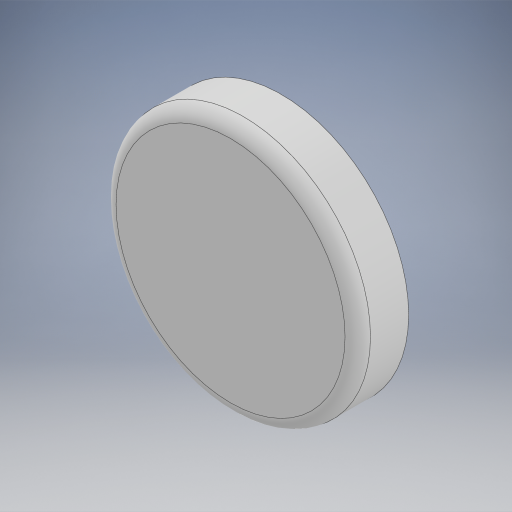
# Autodesk Inventor part: Brikker
Saved by Autodesk Inventor 2024 (Build 280153000, 153)
## iProperties
Created: 2024-03-15
Part Number: Brikker
Material: Generic
Document SubType Name: Modeling
Designer: fluen
Density: 1 g/cm^3
Appearance: Default
Author: fluen
## iProperties of the stored document Brikker_3DPrint.ipt
Created: 2024-04-12
Part Number: Brikker_3DPrint
Material: Generic
Document SubType Name: Modeling
Designer: Faber
Density: 1 g/cm^3
Appearance: Default
Author: Faber
Autodesk Inventor part; units mm, degrees
ref_plane "YZ Plane" through (0, 0, 0) normal (1, 0, 0) x (0, 1, 0)
ref_plane "XZ Plane" through (0, 0, 0) normal (0, 1, 0) x (-1, 0, 0)
ref_plane "XY Plane" through (0, 0, 0) normal (0, 0, 1) x (1, 0, 0)
sketch "Sketch1" plane through (0, 0, 0) normal (0, 0, 1) x (1, 0, 0)
  circle A0 centre (0, 0) radius 10
  dimension "d0" = 20
  constraints: 1 centre point, 1 coincident
  measures "d0" diameter of A0
extrude "Extrusion1" add sketch "Sketch1" along normal mid plane 4
fillet "Fillet1" radius 1 1 edges at (-10, 0, 2)
body "Solid1"
